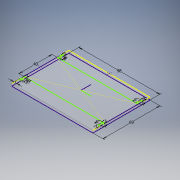
# Autodesk Inventor part: roof_v2
Saved by Autodesk Inventor 2017.2 (Build 212233000, 233)
## iProperties
Created: 2017-06-10
Part Number: roof_v2
Material: Generic
Document SubType Name: Modeling
Designer: SandeepSH
Density: 1 g/cm^3
Appearance: Polycarbonate - Clear
Author: SandeepSH
Autodesk Inventor part; units mm, degrees
ref_plane "YZ Plane" through (0, 0, 0) normal (1, 0, 0) x (0, 1, 0)
ref_plane "XZ Plane" through (0, 0, 0) normal (0, 1, 0) x (-1, 0, 0)
ref_plane "XY Plane" through (0, 0, 0) normal (0, 0, 1) x (1, 0, 0)
sketch "Sketch1" plane through (0, 0, 0) normal (0, 1, 0) x (-1, 0, 0)
  line L0 (0, 0) -> (-98, 0)
  line L1 (-98, 0) -> (-98, -69)
  line L2 (-98, -69) -> (0, -69)
  line L3 (0, -69) -> (0, 0)
  dimension "d0" = 98
  dimension "d1" = 69
  constraints: 8 end point, 2 parallel, 1 horizontal, 1 perpendicular
  measures "d0" distance of L2.end L1.end
  measures "d1" distance of L1.end L0.end
extrude "Extrusion1" add sketch "Sketch1" along normal blind 3
sketch "Sketch2" plane through (0, 3, 0) normal (0, 1, 0) x (1, 0, 0)
  line L0 (0, 69) -> (0, 0) projected
  line L1 (0, 37) -> (9.5, 37)
  line L2 (9.5, 37) -> (9.5, 21)
  line L3 (9.5, 21) -> (0, 21)
  line L4 (0, 21) -> (0, 37)
  line L5 (98, 69) -> (0, 69) projected
  line L6 (57, 59.7224) -> (57, 18.4065)
  line L7 (114, 37) -> (104.5, 37)
  line L8 (104.5, 37) -> (104.5, 21)
  line L9 (104.5, 21) -> (114, 21)
  line L10 (114, 21) -> (114, 37)
  point P0 (9.5, 29)
  point P1 (104.5, 29)
  dimension "d4" = 9.5
  dimension "d5" = 16
  dimension "d6" = 8
  dimension "d7" = 40
  dimension "d8" = 57
  constraints: 18 end point, 5 symmetric about line, 2 midpoint, 2 parallel, 1 horizontal, 1 perpendicular, 1 point on line, 1 vertical
  measures "d4" distance of L2.end L3.end
  measures "d5" distance of L1.end L2.end
  measures "d6" distance from line of L1 point (9.5, 29)
  measures "d7" distance from line of L5 point (9.5, 29)
  measures "d8" distance between parallel lines of L0 L6
sketch "Sketch3" plane through (0, 3, 0) normal (0, 1, 0) x (1, 0, 0)
  point P0 (0, 0)
sketch "Sketch4" plane through (0, 3, 0) normal (0, 1, 0) x (1, 0, 0)
  line L0 (9.5, 9.5) -> (104.5, 9.5)
  line L1 (104.5, 9.5) -> (104.5, 48.5)
  line L2 (104.5, 48.5) -> (9.5, 48.5)
  line L3 (9.5, 48.5) -> (9.5, 9.5)
  line L4 (98, 69) -> (0, 69) projected
  line L5 (14.5, 14) -> (99.5, 14)
  line L6 (99.5, 14) -> (99.5, 44)
  line L7 (99.5, 44) -> (14.5, 44)
  line L8 (14.5, 44) -> (14.5, 14)
  line L9 (98, 0) -> (98, 69) projected
  line L10 (104.5, 31) -> (104.5, 47) projected
  point P0 (0, 0)
  point P1 (1.7335, 29)
  point P2 (81.752, 29)
  point P3 (14.5, 29)
  point P4 (57, 14)
  point P5 (41, 5.8312)
  point P6 (114, 31)
  point P7 (57, 48.3096)
  point P8 (57, 9.5)
  dimension "d11" = 95
  dimension "d12" = 39
  dimension "d13" = 40
  dimension "d14" = 19.5
  dimension "d15" = 40
  dimension "d16" = 85
  dimension "d17" = 30
  dimension "d18" = 15
  dimension "d19" = 40
  dimension "d43" = 57
  dimension "d44" = 47.5
  dimension "d45" = 47.5
  dimension "d46" = 47.5
  constraints: 16 end point, 4 parallel, 3 midpoint, 2 horizontal, 2 perpendicular, 1 other
  measures "d11" distance of L2.end L1.end
  measures "d12" distance of L1.end L0.end
  measures "d13" distance from line of L4 point (1.733, 29)
  measures "d14" distance from line of L2 point (81.752, 29)
  measures "d15" distance from line of L4 point (81.752, 29)
  measures "d16" distance of L7.end L6.end
  measures "d17" distance of L6.end L5.end
  measures "d18" distance from line of L7 point (14.5, 29)
  measures "d19" distance from line of L4 point (14.5, 29)
  measures "d44" distance from line of L1 point (57, 48.31)
  measures "d45" distance from line of L10 point (57, 14)
  measures "d46" distance from line of L10 point (57, 9.5)
sketch "Sketch5" plane through (0, 3, 0) normal (0, 1, 0) x (1, 0, 0)
  line L0 (59.5, 9.5) -> (54.5, 9.5)
  line L1 (54.5, 9.5) -> (54.5, 6.5)
  line L2 (54.5, 6.5) -> (59.5, 6.5)
  line L3 (59.5, 6.5) -> (59.5, 9.5)
  line L4 (59.5, 9.5) -> (54.5, 6.5) construction
  line L5 (54.5, 9.5) -> (59.5, 6.5) construction
  line L6 (9.5, 9.5) -> (104.5, 9.5) projected
  line L7 (59.5, 48.5) -> (54.5, 48.5)
  line L8 (54.5, 48.5) -> (54.5, 51.5)
  line L9 (54.5, 51.5) -> (59.5, 51.5)
  line L10 (59.5, 51.5) -> (59.5, 48.5)
  line L11 (59.5, 48.5) -> (54.5, 51.5) construction
  line L12 (54.5, 48.5) -> (59.5, 51.5) construction
  line L13 (104.5, 48.5) -> (9.5, 48.5) projected
  point P0 (0, 0)
  point P1 (57, 8)
  point P2 (57, 50)
  dimension "d23" = 5
  dimension "d24" = 3
  dimension "d25" = 5
  dimension "d26" = 3
  constraints: 24 end point, 4 midpoint, 4 parallel, 2 collinear, 2 horizontal, 2 perpendicular
  measures "d23" distance of L2.end L1.end
  measures "d24" distance of L1.end L0.end
  measures "d25" distance of L8.end L9.end
  measures "d26" distance of L7.end L8.end
sketch "Sketch6" plane through (0, 3, 0) normal (0, 1, 0) x (1, 0, 0)
  line L0 (59.5895, 38.8648) -> (53.5895, 38.8648)
  line L1 (53.5895, 38.8648) -> (53.5895, 48.8648)
  line L2 (53.5895, 48.8648) -> (59.5895, 48.8648)
  line L3 (59.5895, 48.8648) -> (59.5895, 38.8648)
  line L4 (59.5895, 38.8648) -> (56.5895, 38.8648)
  line L5 (56.5895, 38.8648) -> (56.5895, 41.3648)
  line L6 (56.5895, 41.3648) -> (59.5895, 41.3648)
  line L7 (59.5895, 41.3648) -> (59.5895, 38.8648)
  line L8 (59.5895, 48.8648) -> (56.5895, 48.8648)
  line L9 (56.5895, 48.8648) -> (56.5895, 46.3648)
  line L10 (56.5895, 46.3648) -> (59.5895, 46.3648)
  line L11 (59.5895, 46.3648) -> (59.5895, 48.8648)
  line L12 (59.5895, 25.9829) -> (53.5895, 25.9829)
  line L13 (53.5895, 25.9829) -> (53.5895, 35.9829)
  line L14 (53.5895, 35.9829) -> (59.5895, 35.9829)
  line L15 (59.5895, 35.9829) -> (59.5895, 25.9829)
  line L16 (59.5895, 25.9829) -> (56.5895, 25.9829)
  line L17 (56.5895, 25.9829) -> (56.5895, 28.4829)
  line L18 (56.5895, 28.4829) -> (59.5895, 28.4829)
  line L19 (59.5895, 28.4829) -> (59.5895, 25.9829)
  line L20 (59.5895, 35.9829) -> (56.5895, 35.9829)
  line L21 (56.5895, 35.9829) -> (56.5895, 33.4829)
  line L22 (56.5895, 33.4829) -> (59.5895, 33.4829)
  line L23 (59.5895, 33.4829) -> (59.5895, 35.9829)
  point P0 (0, 0)
  dimension "d29" = 6
  dimension "d30" = 10
  dimension "d31" = 3
  dimension "d32" = 2.5
  dimension "d33" = 3
  dimension "d34" = 2.5
  dimension "d35" = 6
  dimension "d36" = 10
  dimension "d37" = 3
  dimension "d38" = 2.5
  dimension "d39" = 3
  dimension "d40" = 2.5
  constraints: 48 end point, 12 parallel, 6 horizontal, 6 perpendicular
  measures "d29" distance of L1.end L2.end
  measures "d30" distance of L0.end L1.end
  measures "d31" distance of L5.end L6.end
  measures "d32" distance of L4.end L5.end
  measures "d33" distance of L10.end L9.end
  measures "d34" distance of L9.end L8.end
  measures "d35" distance of L13.end L14.end
  measures "d36" distance of L12.end L13.end
  measures "d37" distance of L17.end L18.end
  measures "d38" distance of L16.end L17.end
  measures "d39" distance of L22.end L21.end
  measures "d40" distance of L21.end L20.end
sketch "Sketch7" plane through (0, 3, 0) normal (0, 1, 0) x (1, 0, 0)
  line L0 (0, 69) -> (0, 0) projected
  line L1 (98, 69) -> (0, 69) projected
  line L2 (98, 54.5) -> (0, 54.5)
  line L3 (0, 54.5) -> (0, 14.5)
  line L4 (0, 14.5) -> (98, 14.5)
  line L5 (98, 14.5) -> (98, 54.5)
  line L6 (98, 54.5) -> (0, 14.5) construction
  line L7 (0, 54.5) -> (98, 14.5) construction
  line L8 (98, 0) -> (98, 69) projected
  line L9 (0, 14.5) -> (3, 14.5)
  line L10 (3, 14.5) -> (3, 8.5)
  line L11 (3, 8.5) -> (0, 8.5)
  line L12 (0, 8.5) -> (0, 14.5)
  line L13 (49, 34.5) -> (49, 46.5013)
  line L14 (49, 34.5) -> (61.4324, 34.5)
  line L15 (0, 54.5) -> (3, 54.5)
  line L16 (3, 54.5) -> (3, 60.5)
  line L17 (3, 60.5) -> (0, 60.5)
  line L18 (0, 60.5) -> (0, 54.5)
  line L19 (98, 54.5) -> (95, 54.5)
  line L20 (95, 54.5) -> (95, 60.5)
  line L21 (95, 60.5) -> (98, 60.5)
  line L22 (98, 60.5) -> (98, 54.5)
  line L23 (98, 14.5) -> (95, 14.5)
  line L24 (95, 14.5) -> (95, 8.5)
  line L25 (95, 8.5) -> (98, 8.5)
  line L26 (98, 8.5) -> (98, 14.5)
  line L27 (0, 55.5) -> (3, 55.5)
  line L28 (3, 55.5) -> (3, 59.5)
  line L29 (3, 59.5) -> (0, 59.5)
  line L30 (0, 59.5) -> (0, 55.5)
  line L31 (0, 55.5) -> (3, 59.5) construction
  line L32 (3, 55.5) -> (0, 59.5) construction
  line L33 (0, 9.5) -> (3, 9.5)
  line L34 (3, 9.5) -> (3, 13.5)
  line L35 (3, 13.5) -> (0, 13.5)
  line L36 (0, 13.5) -> (0, 9.5)
  line L37 (0, 9.5) -> (3, 13.5) construction
  line L38 (3, 9.5) -> (0, 13.5) construction
  line L39 (95, 55.5) -> (98, 55.5)
  line L40 (98, 55.5) -> (98, 59.5)
  line L41 (98, 59.5) -> (95, 59.5)
  line L42 (95, 59.5) -> (95, 55.5)
  line L43 (95, 55.5) -> (98, 59.5) construction
  line L44 (98, 55.5) -> (95, 59.5) construction
  line L45 (95, 9.5) -> (98, 9.5)
  line L46 (98, 9.5) -> (98, 13.5)
  line L47 (98, 13.5) -> (95, 13.5)
  line L48 (95, 13.5) -> (95, 9.5)
  line L49 (95, 9.5) -> (98, 13.5) construction
  line L50 (98, 9.5) -> (95, 13.5) construction
  point P0 (0, 34.5)
  point P1 (49, 69)
  point P2 (1.5, 57.5)
  point P3 (1.5, 11.5)
  point P4 (96.5, 57.5)
  point P5 (96.5, 11.5)
  dimension "d47" = 40
  dimension "d48" = 3
  dimension "d49" = 6
  dimension "d50" = 6
  dimension "d51" = 3
  dimension "d52" = 6
  dimension "d53" = 3
  dimension "d54" = 6
  dimension "d55" = 3
  dimension "d56" = 3
  dimension "d57" = 4
  dimension "d58" = 3
  dimension "d59" = 4
  dimension "d60" = 3
  dimension "d61" = 4
  dimension "d62" = 3
  dimension "d63" = 4
  constraints: 96 end point, 18 parallel, 12 midpoint, 10 horizontal, 9 perpendicular, 2 collinear, 1 vertical
  measures "d47" distance of L3.end L2.end
  measures "d48" distance of L10.end L11.end
  measures "d49" distance of L9.end L10.end
  measures "d50" distance of L16.end L15.end
  measures "d51" distance of L20.end L21.end
  measures "d52" distance of L19.end L20.end
  measures "d53" distance of L25.end L24.end
  measures "d54" distance of L24.end L23.end
  measures "d55" distance between parallel lines of L16 L18
  measures "d56" distance of L29.end L28.end
  measures "d57" distance of L28.end L27.end
  measures "d58" distance of L35.end L34.end
  measures "d59" distance of L34.end L33.end
  measures "d60" distance of L41.end L40.end
  measures "d61" distance of L40.end L39.end
  measures "d62" distance of L47.end L46.end
  measures "d63" distance of L46.end L45.end
extrude "Extrusion6" cut sketch "Sketch7" against normal through all contours L29 L16 L27 L0 | L8 L39 L20 L41 | L35 L10 L33 L0 | L8 L45 L24 L47
equation "\"d6\" = 0.5 * d5"
equation "\"d14\" = 0.5 * d12"
equation "\"d15\" = d13"
equation "\"d18\" = 0.5 * d17"
equation "\"d19\" = d13"
equation "\"d46\" = d45"
body "Solid1"
